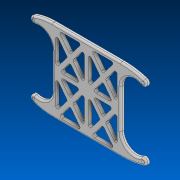
# Autodesk Inventor part: Elevator Tension V2
Saved by Autodesk Inventor 2022 (Build 260153000, 153)
## iProperties
Created: 2022-04-19
Part Number: Elevator Tension V2
Material: Generic
Document SubType Name: Modeling
Designer: score_nygvs6w
Density: 1 g/cm^3
Appearance: Default
Author: score_nygvs6w
Autodesk Inventor part; units mm, degrees
ref_plane "YZ Plane" through (0, 0, 0) normal (1, 0, 0) x (0, 1, 0)
ref_plane "XZ Plane" through (0, 0, 0) normal (0, 1, 0) x (-1, 0, 0)
ref_plane "XY Plane" through (0, 0, 0) normal (0, 0, 1) x (1, 0, 0)
sketch "Sketch1" plane through (0, 0, 0) normal (0, 0, 1) x (1, 0, 0)
  line L0 (63.5, 76.2) -> (-63.5, 76.2)
  line L1 (-63.5, 76.2) -> (-63.5, -76.2)
  line L2 (-63.5, -76.2) -> (63.5, -76.2)
  line L3 (63.5, -76.2) -> (63.5, 76.2)
  line L4 (63.5, 76.2) -> (-63.5, -76.2) construction
  line L5 (-63.5, 76.2) -> (63.5, -76.2) construction
  line L6 (-57.15, 69.85) -> (57.15, 69.85)
  line L7 (57.15, 69.85) -> (57.15, -69.85)
  line L8 (57.15, -69.85) -> (-57.15, -69.85)
  line L9 (-57.15, -69.85) -> (-57.15, 69.85)
  line L10 (-3.81, -69.85) -> (-3.81, 69.85)
  line L11 (3.81, 69.85) -> (3.81, -69.85)
  line L12 (0, 69.85) -> (0, -69.85) construction
  line L13 (-57.15, -69.85) -> (-3.81, 0) construction
  line L14 (-3.81, 0) -> (-57.15, 69.85) construction
  line L15 (3.81, 0) -> (57.15, 69.85) construction
  line L16 (3.81, 0) -> (57.15, -69.85) construction
  line L17 (3.81, -6.2777) -> (52.3561, -69.85)
  line L18 (57.15, -63.5723) -> (6.2069, 3.1388)
  line L19 (3.81, -6.2777) -> (57.15, 63.5723)
  line L20 (52.3561, 69.85) -> (3.81, 6.2777)
  line L21 (-3.81, 6.2777) -> (-52.3561, 69.85)
  line L22 (-57.15, 63.5723) -> (-3.81, -6.2777)
  line L23 (-3.81, 6.2777) -> (-57.15, -63.5723)
  line L24 (-52.3561, -69.85) -> (-3.81, -6.2777)
  line L25 (-57.15, 0) -> (-3.81, 69.85) construction
  line L26 (3.81, 69.85) -> (57.15, 0) construction
  line L27 (57.15, 0) -> (3.81, -69.85) construction
  line L28 (-3.81, -69.85) -> (-57.15, 0) construction
  line L29 (-6.8381, -72.1623) -> (-60.1781, -2.3123)
  line L30 (-60.1781, -2.3123) -> (-54.1219, 2.3123)
  line L31 (-54.1219, 2.3123) -> (-0.7819, -67.5377)
  line L32 (-0.7819, -67.5377) -> (-6.8381, -72.1623)
  line L33 (-6.8381, -72.1623) -> (-54.1219, 2.3123) construction
  line L34 (-60.1781, -2.3123) -> (-0.7819, -67.5377) construction
  line L35 (-54.1219, -2.3123) -> (-0.7819, 67.5377)
  line L36 (-0.7819, 67.5377) -> (-6.8381, 72.1623)
  line L37 (-6.8381, 72.1623) -> (-60.1781, 2.3123)
  line L38 (-60.1781, 2.3123) -> (-54.1219, -2.3123)
  line L39 (-54.1219, -2.3123) -> (-6.8381, 72.1623) construction
  line L40 (-0.7819, 67.5377) -> (-60.1781, 2.3123) construction
  line L41 (54.1219, -2.3123) -> (0.7819, 67.5377)
  line L42 (0.7819, 67.5377) -> (6.8381, 72.1623)
  line L43 (6.8381, 72.1623) -> (60.1781, 2.3123)
  line L44 (60.1781, 2.3123) -> (54.1219, -2.3123)
  line L45 (54.1219, -2.3123) -> (6.8381, 72.1623) construction
  line L46 (0.7819, 67.5377) -> (60.1781, 2.3123) construction
  line L47 (54.1219, 2.3123) -> (0.7819, -67.5377)
  line L48 (0.7819, -67.5377) -> (6.8381, -72.1623)
  line L49 (6.8381, -72.1623) -> (60.1781, -2.3123)
  line L50 (60.1781, -2.3123) -> (54.1219, 2.3123)
  line L51 (54.1219, 2.3123) -> (6.8381, -72.1623) construction
  line L52 (0.7819, -67.5377) -> (60.1781, -2.3123) construction
  line L53 (-3.81, 3.81) -> (-49.4467, 3.81)
  line L54 (-49.4467, 3.81) -> (-49.4467, -3.81)
  line L55 (-49.4467, -3.81) -> (-3.81, -3.81)
  line L56 (-3.81, -3.81) -> (-3.81, 3.81)
  line L57 (-3.81, 3.81) -> (-49.4467, -3.81) construction
  line L58 (-49.4467, 3.81) -> (-3.81, -3.81) construction
  line L59 (3.81, 3.81) -> (49.4467, 3.81)
  line L60 (49.4467, 3.81) -> (49.4467, -3.81)
  line L61 (49.4467, -3.81) -> (3.81, -3.81)
  line L62 (3.81, -3.81) -> (3.81, 3.81)
  line L63 (3.81, 3.81) -> (49.4467, -3.81) construction
  line L64 (49.4467, 3.81) -> (3.81, -3.81) construction
  circle A0 centre (104.9549, 63.5) radius 6.35
  circle A1 centre (-98.2451, 63.5) radius 6.35
  circle A2 centre (-98.2451, -63.5) radius 6.35
  circle A3 centre (104.9549, -63.5) radius 6.35
  line L65 (-63.5, 0) -> (63.5, 0) construction
  arc A4 (101.7439, 58.0217) -> (63.5, 36.1083) centre (88.9, 36.1083) ccw
  arc A5 (63.5, -36.1083) -> (101.7439, -58.0217) centre (88.9, -36.1083) ccw
  arc A6 (-96.3761, -57.4313) -> (-63.5, -33.1565) centre (-88.9, -33.1565) ccw
  arc A7 (-63.5, 33.1565) -> (-96.3761, 57.4313) centre (-88.9, 33.1565) ccw
  arc A8 (-63.5, 76.2) -> (-100.4912, 69.4395) centre (-63.5, -28.3821) ccw
  arc A9 (-100.4912, -69.4395) -> (-63.5, -76.2) centre (-63.5, 28.3821) ccw
  arc A10 (63.5, -76.2) -> (106.8556, -69.5588) centre (63.5, 68.6404) ccw
  arc A11 (106.8556, 69.5588) -> (63.5, 76.2) centre (63.5, -68.6404) ccw
  point P0 (0, 0)
  point P1 (-30.48, -34.925)
  point P2 (-30.48, 34.925)
  point P3 (30.48, 34.925)
  point P4 (30.48, -34.925)
  point P5 (-26.6283, 0)
  point P6 (26.6283, 0)
  point P7 (-26.6283, 0)
  point P8 (0, 0)
  point P9 (26.6283, 0)
  point P10 (0, 0)
  point P11 (25.6861, -34.925)
  point P12 (3.81, -63.5723)
  point P13 (-8.6039, 69.85)
  point P14 (-30.48, 41.2027)
  point P15 (-11.5133, -3.81)
  point P16 (-30.48, -28.6473)
  point P17 (-50.6841, -3.175)
  point P18 (25.6861, 34.925)
  point P19 (3.81, 63.5723)
  point P20 (30.48, 41.2027)
  point P21 (8.6039, 69.85)
  point P22 (30.48, -41.2027)
  point P23 (8.6039, -69.85)
  point P24 (-25.6861, -34.925)
  point P25 (-3.81, -63.5723)
  point P26 (-35.2739, 34.925)
  point P27 (-57.15, 6.2777)
  point P28 (35.2739, -34.925)
  point P29 (57.15, -6.2777)
  point P30 (30.48, -28.6473)
  point P31 (11.5133, -3.81)
  point P32 (50.6841, -3.175)
  point P33 (35.2739, 34.925)
  point P34 (57.15, 6.2777)
  point P35 (30.48, 28.6473)
  point P36 (49.4467, 3.81)
  point P37 (11.5133, 3.81)
  point P38 (-49.4467, 3.81)
  point P39 (-30.48, 28.6473)
  point P40 (-11.5133, 3.81)
  point P41 (-30.48, -41.2027)
  point P42 (-8.6039, -69.85)
  point P43 (-35.2739, -34.925)
  point P44 (-57.15, -6.2777)
  point P45 (-3.81, 63.5723)
  point P46 (-25.6861, 34.925)
  point P47 (63.5, 63.5)
  point P48 (63.5, -63.5)
  point P49 (-63.5, -63.5)
  point P50 (-63.5, 63.5)
  dimension "d0" = 127
  dimension "d1" = 152.4
  dimension "d4" = 6.35
  dimension "d5" = 3.81
  dimension "d6" = 3.81
  dimension "d7" = 3.81
  dimension "d8" = 3.81
  dimension "d9" = 3.81
  dimension "d10" = 3.81
  dimension "d30" = 12.7
  dimension "d38" = 127
  dimension "d39" = 63.5
  dimension "d41" = 203.2
  dimension "d42" = 25.4
  constraints: 132 end point, 35 midpoint, 32 parallel, 26 point on line, 24 point on circle, 16 tangent, 12 centre point, 11 perpendicular, 6 equal radius, 5 equal length, 5 horizontal alignment, 4 coincident, 2 collinear, 2 horizontal, 2 vertical alignment, 8 other
  measures "d0" distance of L0.start L0.end
  measures "d1" distance between parallel lines of L2 L0
  measures "d4" distance between parallel lines of L0 L6
  measures "d5" distance between parallel lines of L12 L10
  measures "d6" distance between parallel lines of L23 L13
  measures "d7" distance between parallel lines of L15 L20
  measures "d8" distance between parallel lines of L16 L18
  measures "d9" distance between parallel lines of L14 L22
  measures "d10" distance between parallel lines of L37 L25
  measures "d30" diameter of A1
  measures "d38" distance of A2.centre A1.centre
  measures "d39" vertical distance of L65.start A2.centre
  measures "d41" distance of point (104.955, 63.5) point (-98.245, 63.5)
  measures "d42" radius of A7
extrude "Extrusion1" add sketch "Sketch1" along normal blind 6.35 contours L3 L2 L1 L0 | A11 A0 A4 L3 | L1 A7 A1 A8 | A0 | A1 | A5 A3 A10 L3 | L1 A9 A2 A6 | A3 | A2 | L6 L21 L37 L22 L9 | L37 L36 L6 | L6 L10 L35 L21 L37 | L21 L35 L22 L37 | L37 L22 L35 L31 L30 L9 | L9 L38 L37 | L36 L35 L10 | L6 L42 L41 L11 L47 L48 L8 L32 L31 L10 L35 L36 | L21 L23 L53 L22 L35 | L38 L35 L31 L23 L29 L9 | L9 L29 L30 | L30 L31 L35 L38 | L42 L43 L6 | L6 L43 L20 L41 L11 | L11 L41 L42 | L10 L53 L23 | L53 L23 L22 | L22 L23 L55 L54 L53 | L54 L31 L35 | L10 L55 L22 L23 L53 | L23 L29 L24 L8 L9 | L23 L31 L24 L29 | L22 L55 L23 | L6 L7 L19 L43 L20 | L43 L19 L41 L20 | L20 L41 L19 L59 L11 | L10 L22 L55 | L23 L55 L22 L24 L31 | L24 L31 L10 L8 L29 | L43 L7 L50 L47 L41 L19 | L59 L19 L61 L11 | L8 L32 L29 | L43 L44 L7 | L61 L19 L11 | L59 L60 L61 L18 L19 | L41 L47 L60 | L31 L32 L10 | L50 L49 L7 | L7 L49 L18 L47 L41 L44 | L44 L41 L47 L50 | L19 L61 L18 L47 L17 | L19 L18 L61 | L11 L47 L17 L49 L8 | L48 L47 L11 | L8 L49 L48 | L47 L18 L49 L17 | L7 L8 L17 L49 L18
fillet "Fillet1" radius 3.175 48 edges at (52.3561, -69.85, 3.175) (57.15, -63.5723, 3.175) (35.2739, -34.925, 3.175) (57.15, -6.2777, 3.175) (49.4467, -3.81, 3.175) (49.4467, 3.81, 3.175) (57.15, 6.2777, 3.175) (30.48, -41.2027, 3.175) (25.6861, -34.925, 3.175) (30.48, -28.6473, 3.175) (8.6039, -69.85, 3.175) (3.81, -63.5723, 3.175) (3.81, -6.2777, 3.175) (11.5133, -3.81, 3.175) (-3.81, -63.5723, 3.175) (-8.6039, -69.85, 3.175) (-30.48, -41.2027, 3.175) (-52.3561, -69.85, 3.175) (-57.15, -63.5723, 3.175) (-35.2739, -34.925, 3.175) (-30.48, -28.6473, 3.175) (-25.6861, -34.925, 3.175) (-3.81, -6.2777, 3.175) (-11.5133, -3.81, 3.175) (-49.4467, -3.81, 3.175) (-57.15, -6.2777, 3.175) (-49.4467, 3.81, 3.175) (-57.15, 6.2777, 3.175) (-11.5133, 3.81, 3.175) (-3.81, 6.2777, 3.175) (3.81, 6.2777, 3.175) (11.5133, 3.81, 3.175) (30.48, 28.6473, 3.175) (35.2739, 34.925, 3.175) (25.6861, 34.925, 3.175) (30.48, 41.2027, 3.175) (57.15, 63.5723, 3.175) (52.3561, 69.85, 3.175) (8.6039, 69.85, 3.175) (3.81, 63.5723, 3.175) (-25.6861, 34.925, 3.175) (-3.81, 63.5723, 3.175) (-8.6039, 69.85, 3.175) (-52.3561, 69.85, 3.175) (-30.48, 41.2027, 3.175) (-30.48, 28.6473, 3.175) (-35.2739, 34.925, 3.175) (-57.15, 63.5723, 3.175)
hole "Hole2" at (-98.2451, 63.5, 0) at (-98.2451, -63.5, 0) at (104.9549, -63.5, 0) at (104.9549, 63.5, 0) direction (0, 0, 1) diameter 4.445 end through all
fillet "Fillet4" radius 3.175 16 edges at (85.4307, -74.5301, 6.35) (110.7605, -60.9277, 6.35) (76.2721, -58.1469, 6.35) (63.5, 0, 6.35) (76.2721, 58.1469, 6.35) (110.7605, 60.9277, 6.35) (85.4307, 74.5301, 6.35) (0, 76.2, 6.35) (-82.3019, 74.496, 6.35) (-104.2522, 61.4415, 6.35) (-73.8125, 53.5899, 6.35) (-63.5, 0, 6.35) (-73.8125, -53.5899, 6.35) (-104.2522, -61.4415, 6.35) (-82.3019, -74.496, 6.35) (0, -76.2, 6.35)
sketch "Sketch2" plane through (-63.5, 76.2, 0) normal (0, 1, 0) x (1, 0, 0)
  line L0 (-25.4, 80.9625) -> (-22.225, 80.9625)
  line L1 (-22.225, 80.9625) -> (-22.225, 55.5625)
  line L2 (-22.225, 55.5625) -> (-25.4, 55.5625)
  line L3 (-25.4, 55.5625) -> (-25.4, 80.9625)
  line L4 (152.4, 80.9625) -> (149.225, 80.9625)
  line L5 (149.225, 80.9625) -> (149.225, 55.5625)
  line L6 (149.225, 55.5625) -> (152.4, 55.5625)
  line L7 (152.4, 55.5625) -> (152.4, 80.9625)
  line L8 (127, -6.35) -> (0, -6.35) projected
  line L9 (63.5, 0) -> (63.5, 80.9625) construction
  line L10 (127, 0) -> (0, 0) projected
  line L11 (0, 0) -> (0, -3.175) projected
  line L12 (127, -3.175) -> (0, -3.175) projected
  line L13 (127, 0) -> (127, -3.175) projected
  line L14 (0, 0) -> (0, -6.35) projected
  line L15 (1.1567, -5.8498) -> (-25.4, 55.5625)
  line L16 (0, 0) -> (127, 0) projected
  line L17 (2.0862, 0) -> (-22.225, 56.2196)
  line L18 (127, 0) -> (127, -6.35) projected
  line L19 (125.8433, -5.8498) -> (152.4, 55.5625)
  line L20 (149.225, 56.2196) -> (124.9138, 0)
  point P0 (2.0862, 0)
  dimension "d12" = 25.4
  dimension "d13" = 58.7375
  dimension "d14" = 3.175
  dimension "d15" = 177.8
  dimension "d16" = 3.175
  dimension "d17" = 3.175
  constraints: 22 end point, 5 point on line, 4 parallel, 2 equal length, 2 horizontal, 2 perpendicular, 1 collinear, 1 vertical, 9 other
  measures "d12" distance of L0.end L1.end
  measures "d14" distance between parallel lines of L3 L1
  measures "d15" distance between parallel lines of L7 L3
sketch "Sketch3" plane through (88.9, 50.8, -56.351) normal (1, 0, 0) x (0, 0, -1)
  arc A0 (11.9115, 0) -> (11.9115, 25.4) centre (11.9115, 12.7) ccw projected
  point P0 (-56.351, -50.8)
  constraints: 1 coincident
equation "\"d6\" = d5"
equation "\"d7\" = d5"
equation "\"d8\" = d7"
equation "\"d9\" = d5"
equation "\"d10\" = d5"
body "Solid1"
